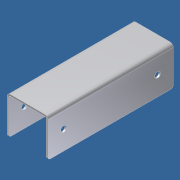
# Autodesk Inventor part: GE-12052_modified
Saved by Autodesk Inventor 2012 (Build 160160000, 160)
## iProperties
Created: 2011-06-20
Part Number: GE-12052_modified
Document SubType Name: Modeling
Designer: dfoster
Density: 1 g/cm^3
Description: Channel, Net Bracket
Material: Default
Title: Channel, Net Bracket
Author: dfoster
Autodesk Inventor part; units mm, degrees
ref_plane "YZ Plane" through (0, 0, 0) normal (1, 0, 0) x (0, 1, 0)
ref_plane "XZ Plane" through (0, 0, 0) normal (0, 1, 0) x (-1, 0, 0)
ref_plane "XY Plane" through (0, 0, 0) normal (0, 0, 1) x (1, 0, 0)
sketch "Sketch1" plane through (0, 0, 0) normal (0, 0, 1) x (1, 0, 0)
  line L0 (0, 0) -> (0, 42.4688)
  line L1 (4.0132, 46.482) -> (45.6692, 46.482)
  line L2 (49.6824, 42.4688) -> (49.6824, 0)
  arc A0 (4.0132, 46.482) -> (0, 42.4688) centre (4.0132, 42.4688) ccw
  arc A1 (49.6824, 42.4688) -> (45.6692, 46.482) centre (45.6692, 42.4688) ccw
  line L3 (47.7012, 0) -> (47.7012, 42.4688)
  arc A2 (47.7012, 42.4688) -> (45.6692, 44.5008) centre (45.6692, 42.4688) ccw
  line L4 (45.6692, 44.5008) -> (4.0132, 44.5008)
  arc A3 (4.0132, 44.5008) -> (1.9812, 42.4688) centre (4.0132, 42.4688) ccw
  line L5 (1.9812, 42.4688) -> (1.9812, 0)
  line L6 (0, 0) -> (1.9812, 0)
  line L7 (47.7012, 0) -> (49.6824, 0)
  dimension "d1" = 1.9812
  dimension "d3" = 46.482
  dimension "d6" = 45.72
  dimension "d7" = 2.032
  constraints: 16 end point, 8 point on circle, 4 centre point, 4 tangent, 3 equal length, 3 perpendicular, 1 equal radius, 1 vertical, 4 other
  measures "d1" distance between parallel lines of L4 L1
  measures "d3" distance between parallel lines of L1 L6
  measures "d6" distance between parallel lines of L3 L5
  measures "d7" radius of A2
extrude "Extrusion1" add sketch "Sketch1" along normal blind 152.4
fillet "Fillet1" radius 3.175 4 edges at (0.9906, 0, 152.4) (48.6918, 0, 152.4) (48.6918, 0, 0) (0.9906, 0, 0)
hole "Hole1" at (49.6824, 23.241, 133.35) direction (-1, 0, 0) diameter 6.985 end through all
pattern_linear "Rectangular Pattern1" count 2 spacing 114.3 along (0, 0, -1) of "Hole1"
body "Solid1"
